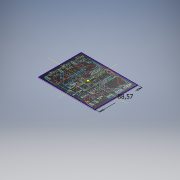
# Autodesk Inventor part: BotControllerPCB
Saved by Autodesk Inventor 2018.3 (Build 223284000, 284)
## iProperties
Created: 2018-08-20
Part Number: BotControllerPCB
Material: Generisch
Document SubType Name: Modeling
Designer: JochenAlt
Density: 1 g/cm^3
Appearance: Vorgabe
Author: JochenAlt
Autodesk Inventor part; units mm, degrees
ref_plane "YZ Plane" through (0, 0, 0) normal (1, 0, 0) x (0, 1, 0)
ref_plane "XZ Plane" through (0, 0, 0) normal (0, 1, 0) x (-1, 0, 0)
ref_plane "XY Plane" through (0, 0, 0) normal (0, 0, 1) x (1, 0, 0)
sketch "Skizze1" plane through (0, 0, 0) normal (0, 0, 1) x (1, 0, 0)
  line L0 (-58.5364, 44.285) -> (58.5364, 44.285)
  line L1 (58.5364, 44.285) -> (58.5364, -44.285)
  line L2 (58.5364, -44.285) -> (-58.5364, -44.285)
  line L3 (-58.5364, -44.285) -> (-58.5364, 44.285)
  line L4 (-81.951, 0) -> (81.951, 0) construction
  line L5 (0, -61.999) -> (0, 61.999) construction
  line L6 (-58.5364, 44.285) -> (58.5364, 44.285) construction
  line L7 (58.5364, 44.285) -> (58.5364, -44.285) construction
  line L8 (58.5364, -44.285) -> (-58.5364, -44.285) construction
  line L9 (-58.5364, -44.285) -> (-58.5364, 44.285) construction
  point P0 (0, 0)
  dimension "d0" = 88.57
  constraints: 8 end point, 3 parallel, 2 point on line, 1 horizontal, 1 perpendicular, 4 other
  measures "d0" distance of L0.end L1.end
extrude "Extrusion1" add sketch "Skizze1" against normal blind 2
